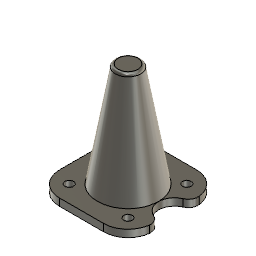
Patas Quadcopter (Autodesk Fusion 360 design; units mm, degrees)
Autodesk Fusion 360 part; units mm, degrees
note: some values were not read from the file. Chosen so that the rebuilt part matches the saved one: which face or edge a step refers to; which pieces of a blend or face edit are solid.
sketch "Boceto1" plane through (0, 0, 0) normal (1, 0, 0) x (0, 1, 0)
  line L0 (0, 0) -> (0, 40)
  line L1 (0, 40) -> (4, 40)
  line L2 (0, 0) -> (12, 0)
  line L3 (12, 0) -> (5.1776, 38.9851)
  arc A0 (5.1776, 38.9851) -> (4, 40) centre (3.9693, 38.7737) ccw
  dimension "d2" = 40
  constraint coincident L0.start L2.start
  constraint perpendicular L0 L1
  constraint perpendicular L0 L2
  constraint tangent L3 A0
  constraint coincident L1 A0.end
  constraint coincident A0 L1.end
  measures "d2" distance of L0.start L0.end
revolve "Revolución2" add sketch "Boceto1" angle 360 about axis through (0, 0, 0) along (0, 0, 1)
sketch "Boceto3" plane through (0, 0, 0) normal (0, 0, -1) x (1, 0, 0)
  circle A0 centre (0, 0) radius 12
  line L0 (-19, 0) -> (-19, -19)
  line L1 (-19, -19) -> (19, -19)
  line L2 (19, -19) -> (19, 19)
  line L3 (19, 19) -> (-19, 19)
  line L4 (-19, 19) -> (-19, 0)
  circle A1 centre (12.0209, -12.0209) radius 1.75
  circle A2 centre (12.0209, 12.0209) radius 1.75
  circle A3 centre (-12.0209, 12.0209) radius 1.75
  circle A4 centre (-12.0209, -12.0209) radius 1.75
  dimension "d20" = 360
  constraint perpendicular L0 L1
  constraint perpendicular L1 L2
  constraint perpendicular L2 L3
extrude "Extruir1" add sketch "Boceto3" along normal blind 2 contours A0 | L0 L1 L2 L3 L4
hole "Hole1" at (19, 0, 0) direction (0, 0, -1) diameter 13 depth 5 tip angle 118
fillet "Fillet1" radius 10 1 edges at (-19, -19, -1)
fillet "Fillet2" radius 10 1 edges at (19, -19, -1)
fillet "Fillet3" radius 10 1 edges at (19, 19, -1)
fillet "Fillet4" radius 10 1 edges at (-19, 19, -1)
fillet "Fillet5" radius 4 1 edges at (19, -6.5, -1)
fillet "Fillet6" radius 4 1 edges at (19, 6.5, -1)
move_face "MoveFace1" to x (1, 0, 0) y (0, 1, 0) z (0, 0, 1) at (0, 0, 2.5) 3 faces at (9.7358, 5.621, 4.3317) (-0.2575, -5.1602, 39.0402) (1.5239, -0.144, 40)
move_face "MoveFace2" by (0, 0, -1) 1 faces at (-3.1198, 0, -2)
revolve "Revolución1" [suppressed]
sketch "Boceto2" plane through (0, 0, 0) normal (0, 0, -1) x (1, 0, 0)
  circle A0 centre (0, 0) radius 15
  line L0 (19, 0) -> (19, -19)
  line L1 (19, -19) -> (19, 19)
  line L2 (19, 19) -> (-19, 19)
  line L3 (-19, 19) -> (-19, -19)
  line L4 (-19, -19) -> (19, -19)
  line L5 (-19, 19) -> (-12.0209, 12.0209)
  circle A1 centre (-12.0209, 12.0209) radius 1.75
  dimension "d7" = 38
  dimension "d10" = 9.87
  dimension "d11" = 3.5
  constraint parallel L0 L1
  constraint perpendicular L1 L2
  constraint perpendicular L2 L3
  constraint coincident L5.end A1.centre
  measures "d7" distance of L0.end L1.end
  measures "d10" distance of L2.end L5.end
  measures "d11" diameter of A1
